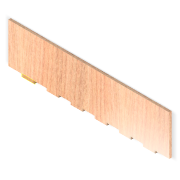
# Autodesk Inventor part: zijkant electronica
Saved by Autodesk Inventor 2020.3 (Build 243373000, 373)
## iProperties
Created: 2020-10-19
Part Number: zijkant electronica
Material: Wood (Birch)
Document SubType Name: Sheet Metal
Designer: Svend
Density: 0.55 g/cm^3
Sheet Metal Rule: Default_mm
Appearance: Birch - Natural Polished
Author: Svend
Autodesk Inventor part; units mm, degrees
ref_plane "YZ Plane" through (0, 0, 0) normal (1, 0, 0) x (0, 1, 0)
ref_plane "XZ Plane" through (0, 0, 0) normal (0, 1, 0) x (-1, 0, 0)
ref_plane "XY Plane" through (0, 0, 0) normal (0, 0, 1) x (1, 0, 0)
ref_plane "Work Plane1" through (0, 0, 0) normal (0, 0, 1) x (1, 0, 0)
sketch "Sketch1" plane through (0, 0, 0) normal (0, 0, 1) x (1, 0, 0)
  line L0 (0, 0) -> (30, 0)
  line L1 (0, 0) -> (0, -6)
  line L2 (30, -6) -> (0, -6)
  line L3 (30, 0) -> (30, -6)
  line L4 (60, 0) -> (90, 0)
  line L5 (60, 0) -> (60, -6)
  line L6 (90, -6) -> (60, -6)
  line L7 (90, 0) -> (90, -6)
  line L8 (120, 0) -> (150, 0)
  line L9 (120, 0) -> (120, -6)
  line L10 (150, -6) -> (120, -6)
  line L11 (150, 0) -> (150, -6)
  line L12 (180, 0) -> (210, 0)
  line L13 (180, 0) -> (180, -6)
  line L14 (210, -6) -> (180, -6)
  line L15 (210, 0) -> (210, -6)
  line L16 (240, 0) -> (270, 0)
  line L17 (240, 0) -> (240, -6)
  line L18 (270, -6) -> (240, -6)
  line L19 (270, 0) -> (270, -6)
  line L20 (300, 0) -> (330, 0)
  line L21 (300, 0) -> (300, -6)
  line L22 (330, -6) -> (300, -6)
  line L23 (330, 0) -> (330, -6)
  line L24 (330, 0) -> (330, -6)
  line L25 (330, -6) -> (365, -6)
  line L26 (365, -6) -> (365, 0)
  line L27 (365, 0) -> (330, 0)
  line L28 (300, -6) -> (300, 0)
  line L29 (300, 0) -> (270, 0)
  line L30 (270, 0) -> (270, -6)
  line L31 (270, -6) -> (300, -6)
  line L32 (210, 0) -> (210, -6)
  line L33 (210, -6) -> (240, -6)
  line L34 (240, -6) -> (240, 0)
  line L35 (240, 0) -> (210, 0)
  line L36 (150, 0) -> (150, -6)
  line L37 (150, -6) -> (180, -6)
  line L38 (180, -6) -> (180, 0)
  line L39 (180, 0) -> (150, 0)
  line L40 (120, -6) -> (120, 0)
  line L41 (120, 0) -> (90, 0)
  line L42 (90, 0) -> (90, -6)
  line L43 (90, -6) -> (120, -6)
  line L44 (30, 0) -> (30, -6)
  line L45 (30, -6) -> (60, -6)
  line L46 (60, -6) -> (60, 0)
  line L47 (60, 0) -> (30, 0)
  line L48 (0, -6) -> (0, 0)
  line L49 (0, 0) -> (-35, 0)
  line L50 (-35, -6) -> (-35, 0)
  line L51 (-35, -6) -> (0, -6)
  line L52 (0, 0) -> (-35, 0)
  line L53 (30, 0) -> (60, 0)
  line L54 (90, 0) -> (120, 0)
  line L55 (150, 0) -> (180, 0)
  line L56 (210, 0) -> (240, 0)
  line L57 (270, 0) -> (300, 0)
  line L58 (330, 0) -> (365, 0)
  line L59 (330, 0) -> (330, -6)
  line L60 (300, 0) -> (300, -6)
  line L61 (330, -6) -> (300, -6)
  line L62 (270, 0) -> (270, -6)
  line L63 (240, -6) -> (240, 0)
  line L64 (240, -6) -> (270, -6)
  line L65 (210, 0) -> (210, -6)
  line L66 (180, -6) -> (210, -6)
  line L67 (180, -6) -> (180, 0)
  line L68 (150, 0) -> (150, -6)
  line L69 (120, -6) -> (150, -6)
  line L70 (120, -6) -> (120, 0)
  line L71 (90, 0) -> (90, -6)
  line L72 (90, -6) -> (60, -6)
  line L73 (60, 0) -> (60, -6)
  line L74 (30, 0) -> (30, -6)
  line L75 (0, 0) -> (0, -6)
  line L76 (30, -6) -> (0, -6)
  line L77 (-35, 0) -> (-35, 100)
  line L78 (-35, 100) -> (365, 100)
  line L79 (365, 0) -> (365, 100)
  dimension "d0" = 100
  measures "d0" distance of L49.end L77.end
extrude "Plate1" add sketch "Sketch1" along normal blind 6 contours L49 L77 L78 L79 L27 L20 L29 L16 L35 L12 L39 L8 L41 L4 L47 L0 | L0 L3 L2 L1 | L4 L7 L6 L5 | L8 L11 L10 L9 | L23 L22 L21 L20 | L12 L15 L14 L13 | L19 L18 L17 L16
equation "\"d1\" = Thickness"
equation "\"BendRadius\" = Thickness"
equation "\"BendReliefWidth\" = Thickness"
equation "\"BendReliefDepth\" = 0.5 * Thickness"
equation "\"CornerReliefSize\" = 4 * Thickness"
equation "\"MinimumRemnant\" = 2 * Thickness"
equation "\"TransitionRadius\" = BendRadius"
equation "\"JacobiRadiusSize\" = BendRadius"
equation "\"GapSize\" = Thickness"
equation "\"Thickness\" = 6"
body "Solid1"
